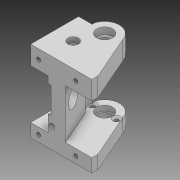
# Autodesk Inventor part: thumb_03 CMC bottom
Saved by Autodesk Inventor 2017 SP1 (Build 210196100, 196)
## iProperties
Created: 2018-02-05
Part Number: thumb_03 CMC bottom
Material: Generic
Document SubType Name: Modeling
Designer: JT
Density: 1 g/cm^3
Appearance: Default
Author: JT
Autodesk Inventor part; units mm, degrees
note: some values were not read from the file. Chosen so that the rebuilt part matches the saved one: direction of "right mount"; direction of "left mount".
sketch3d "geometry"
ref_plane "right inside" through (0, 0, 7.5) normal (0, 0, 1) x (1, 0, 0)
ref_plane "left inside" through (0, 0, -11) normal (0, 0, 1) x (1, 0, 0)
ref_plane "middle top" through (-7.2233, 5.2986, 0) normal (-0.916472, -0.4000988, 0) x (0.4000988, -0.916472, 0)
sketch "Sketch1" plane through (0, 0, 7.5) normal (0, 0, 1) x (1, 0, 0)
  line L0 (-18, 0) -> (5, 0)
  line L1 (5, 0) -> (5, 19)
  line L2 (5, 19) -> (-18, 19)
  line L3 (-18, 19) -> (-18, 0)
  circle A0 centre (-7.6003, 17.4093) radius 5.5
  point P0 (0, 0)
  point P1 (0, 18)
  dimension "d12" = 18
  dimension "d13" = 5
  dimension "d69" = 1
  dimension "d150" = 11
  constraints: 8 end point, 2 parallel, 1 centre point, 1 coincident, 1 horizontal, 1 perpendicular, 1 point on line
  measures "d12" distance from line of point (0, 0) L3
  measures "d13" distance from line of L1 point (0, 0)
  measures "d69" distance from line of L2 point (0, 18)
  measures "d150" diameter of A0
extrude "right" add sketch "Sketch1" along normal blind 7
sketch "Sketch2" plane through (0, 0, -11) normal (0, 0, 1) x (1, 0, 0)
  line L0 (5, 0) -> (-18, 0)
  line L1 (-18, 0) -> (-18, 19)
  line L2 (-18, 19) -> (5, 19)
  line L3 (5, 19) -> (5, 0)
  circle A0 centre (-7.6003, 17.4093) radius 5.5
  point P0 (0, 0)
  point P1 (0, 18)
  dimension "d16" = 18
  dimension "d17" = 5
  dimension "d70" = 1
  dimension "d151" = 11
  constraints: 8 end point, 2 parallel, 1 centre point, 1 coincident, 1 horizontal, 1 perpendicular, 1 point on line
  measures "d16" distance from line of L1 point (0, 0)
  measures "d17" distance from line of point (0, 0) L3
  measures "d70" distance from line of L2 point (0, 18)
  measures "d151" diameter of A0
extrude "left" add sketch "Sketch2" against normal blind 5
sketch "Sketch11" plane through (0, 0, -11) normal (0, 0, 1) x (1, 0, 0)
  line L0 (-0.8483, -9.3042) -> (-15.9776, 25.3514) projected
  line L1 (-12.7683, 18) -> (-19.3151, 18)
  line L2 (-19.3151, 18) -> (-11.457, 0)
  line L3 (-11.457, 0) -> (-4.9101, 0)
  point P0 (0, 0)
  point P1 (0, 18)
  dimension "d66" = 6
  constraints: 6 end point, 4 point on line, 2 parallel, 1 horizontal
  measures "d66" distance between parallel lines of L0 L2
extrude "Extrusion4" add sketch "Sketch11" along normal up to surface (18.5 mm away)
sketch "Sketch4" plane through (0, 0, 7.5) normal (0, 0, 1) x (1, 0, 0)
  point P0 (0, 0)
  point P1 (-7.6003, 17.4093)
hole "thrust bearing pocket" at (-7.6003, 17.4093, 7.5) direction (0, 0, 1) diameter 8.5 depth 3.5
sketch "Sketch7" plane through (0, 0, 7.5) normal (0, 0, 1) x (1, 0, 0)
  point P0 (0, 0)
  point P1 (-7.6003, 17.4093)
hole "worm shaft R" at (-7.6003, 17.4093, 7.5) direction (0, 0, 1) diameter 3.5 end through all
sketch "Sketch5" plane through (0, 0, -11) normal (0, 0, 1) x (1, 0, 0)
  point P0 (0, 0)
  point P1 (-7.6003, 17.4093)
hole "worm shaft L" at (-7.6003, 17.4093, -11) direction (0, 0, -1) diameter 5 end through all counterbore diameter 6 counterbore depth 2
sketch "Sketch6" plane through (-7.2233, 5.2986, 0) normal (-0.916472, -0.4000988, 0) x (0.4000988, -0.916472, 0)
  point P0 (7.746, 0)
  point P1 (0, 0)
hole "CMC bearing" at (-7.2233, 5.2986, 0) direction (-0.916472, -0.4000988, 0) diameter 5 end through all counterbore diameter 7 counterbore depth 2.5
sketch "Sketch9" plane through (0, 0, 14.5) normal (0, 0, 1) x (1, 0, 0)
  point P0 (0, 0)
  point P1 (-7.6003, 17.4093)
hole "Hole5" at (-7.6003, 17.4093, 14.5) direction (0, 0, -1) diameter 6 depth 2.5
ref_plane "clearance angular cut" through (1.9414, 9.2995, 0) normal (-0.916472, -0.4000988, 0) x (0.4000988, -0.916472, 0)
ref_plane "Work Plane4" through (-3.0992, 7.099, 0) normal (-0.916472, -0.4000988, 0) x (0.4000988, -0.916472, 0)
sketch "Sketch12" plane through (0, 0, -11) normal (0, 0, 1) x (1, 0, 0)
  circle A0 centre (-7.6003, 17.4093) radius 5.25
  point P0 (0, 0)
  dimension "d71" = 10.5
  constraints: 1 centre point, 1 coincident
  measures "d71" diameter of A0
extrude "worm cutout" cut sketch "Sketch12" along normal up to surface (18.5 mm away)
sketch "Sketch13" plane through (1.9414, 9.2995, 0) normal (-0.916472, -0.4000988, 0) x (0.4000988, -0.916472, 0)
  line L0 (0, 0) -> (10, 0) construction
  line L1 (0, -25) -> (10, -25)
  line L2 (10, 25) -> (0, 25)
  arc A0 (0, 25) -> (0, -25) centre (0, 0) ccw
  arc A1 (10, -25) -> (10, 25) centre (10, 0) ccw
  point P0 (7.746, 0)
  point P1 (5, 0)
  dimension "d74" = 50
  dimension "d75" = 10
  constraints: 8 end point, 4 point on circle, 4 tangent, 2 centre point, 1 horizontal, 1 midpoint, 1 parallel
  measures "d74" diameter of A1
  measures "d75" horizontal distance of L1.end L0.start
extrude "Extrusion6" cut sketch "Sketch13" against normal through all
ref_plane "Work Plane6" through (3.7744, 10.0997, 0) normal (-0.916472, -0.4000988, 0) x (0.4000988, -0.916472, 0)
split "Split2" [suppressed]
sketch "Sketch14" plane through (-18, 19, -11) normal (0, 1, 0) x (1, 0, 0)
  line L0 (15.7066, 0) -> (15.7066, 5) projected
  line L1 (15.6647, 5) -> (15.7066, 5) projected
  line L2 (0, 0) -> (0, 5) projected
  line L3 (0, -18.5) -> (0, -25.5) projected
  line L4 (5.1348, -25.5) -> (0, -25.5) projected
  line L5 (4.3997, 5) -> (4.3997, 0)
  line L6 (4.3997, -18.5) -> (4.3997, -25.5)
  line L7 (15.7066, -18.5) -> (15.6647, -18.5) projected
  line L8 (5.1348, -18.5) -> (5.1348, -25.5) projected
  line L9 (5.1348, -18.5) -> (0, -18.5) projected
  line L10 (15.7066, -25.5) -> (15.7066, -18.5) projected
  line L11 (15.6647, -25.5) -> (15.6647, -18.5) projected
  line L12 (15.6647, 0) -> (15.7066, 0) projected
  line L13 (5.1348, 5) -> (5.1348, 0) projected
  line L14 (15.6647, 0) -> (15.6647, 5) projected
  line L15 (15.7066, -25.5) -> (15.6647, -25.5) projected
  line L16 (0, 5) -> (5.1348, 5) projected
  line L17 (0, 0) -> (5.1348, 0) projected
  point P0 (18, -11)
  point P1 (10.3997, -11)
  dimension "d80" = 6
  constraints: 4 end point, 2 point on line, 1 collinear
  measures "d80" distance from line of point (10.4, -11) L5
extrude "top cutout" cut sketch "Sketch14" against normal up to surface (1 mm away) contours L2 L16 L5 L17 | L5 L16 L13 L17 | L9 L6 L4 L3 | L9 L8 L4 L6
sketch "Sketch15" plane through (0, 0, -11) normal (0, 0, 1) x (1, 0, 0)
  line L0 (-12.1003, 17.4093) -> (-3.1003, 17.4093) construction
  point P0 (0, 0)
  point P1 (-7.6003, 17.4093)
  point P2 (-7.6003, 17.4093)
  dimension "d83" = 9
  constraints: 2 end point, 1 coincident, 1 horizontal, 1 midpoint
  measures "d83" distance of L0.end L0.start
hole "motor mount" at (-12.1003, 17.4093, -11) at (-3.1003, 17.4093, -11) direction (0, 0, -1) diameter 1.6 end through all countersink diameter 3 countersink angle 90
sketch "Sketch16" plane through (-19.3151, 18, -11) normal (0, 1, 0) x (1, 0, 0)
  line L0 (6.4982, -18.5) -> (6.4982, 0) projected
  line L1 (5.8361, 0) -> (6.4982, 0) projected
  line L2 (1.3151, 5) -> (6.4499, 5) projected
  line L3 (1.3151, 0) -> (1.3151, 5) projected
  line L4 (0, 0) -> (1.3151, 0) projected
  line L5 (0, 0) -> (0, -18.5) projected
  line L6 (0, -18.5) -> (1.3151, -18.5) projected
  line L7 (1.3151, -25.5) -> (1.3151, -18.5) projected
  line L8 (6.4499, -25.5) -> (1.3151, -25.5) projected
  line L9 (6.4982, -18.5) -> (6.4499, -18.5) projected
  line L10 (1.3151, 2.5) -> (5.7149, 2.5) construction
  line L11 (1.3151, -22) -> (5.7149, -22) construction
  line L12 (0, -9.25) -> (6.4982, -9.25) construction
  line L13 (6.4499, -18.5) -> (6.4499, -25.5) projected
  line L14 (6.4499, 5) -> (6.4499, 0.5335) projected
  point P0 (19.3151, -11)
  point P1 (3.515, 2.5)
  point P2 (4.9982, -2.75)
  point P3 (4.9982, -15.75)
  point P4 (3.515, -22)
  point P5 (3.515, 2.5)
  point P6 (3.515, -22)
  dimension "d91" = 1.5
  dimension "d92" = 13
  constraints: 6 end point, 6 midpoint, 2 coincident, 1 symmetric about line, 1 other
  measures "d91" distance from line of L0 point (4.998, -2.75)
  measures "d92" distance of point (4.998, -15.75) point (4.998, -2.75)
hole "top mount" at (-15.8001, 18, -13.5) at (-15.8001, 18, 11) direction (0, -1, 0) diameter 1.567 depth 6.3 tip angle 118 thread size "M2x0.4" class "6H" standard "ANSI Metric M Profile"
sketch "Sketch25" plane through (-19.3151, 18, -11) normal (0, 1, 0) x (1, 0, 0)
  point P0 (19.3151, -11)
  point P1 (4.9982, -15.75)
  point P2 (4.9982, -2.75)
hole "top mount screws" at (-14.3169, 18, 4.75) at (-14.3169, 18, -8.25) direction (0, -1, 0) diameter 2 depth 5
sketch "Sketch17" plane through (0, 0, 14.5) normal (0, 0, 1) x (1, 0, 0)
  line L0 (-0.5303, -10.0324) -> (-17.8852, 29.7208) projected
  line L1 (-14.2665, 16.4331) -> (-8.2335, 2.6139) construction
  point P0 (0, 0)
  point P1 (0, 18)
  point P2 (-11.0215, 9)
  dimension "d100" = 2
  dimension "d101" = 9
  constraints: 2 end point, 1 parallel, 1 point on line
  measures "d100" distance between parallel lines of L0 L1
  measures "d101" vertical distance of point (-11.021, 9) point (0, 18)
hole "right mount" at (-11.0215, 9, 14.5) direction (0, 0, -1) diameter 2.2 depth 7 counterbore diameter 4 counterbore depth 2
sketch "Sketch18" plane through (0, 0, -16) normal (0, 0, -1) x (-1, 0, 0)
  line L0 (4.9101, 0) -> (10.6425, 13.1306) projected
  line L1 (10.6425, 13.1306) -> (4.9101, 0) projected
  line L2 (5.8229, 2.0909) -> (8.6236, 8.5062) projected
  line L3 (4.9157, -4.986) -> (12.5315, 12.4589) construction
  point P0 (0, 0)
  point P1 (11.0215, 9)
  point P2 (0, 18)
  dimension "d110" = 2
  dimension "d111" = 9
  constraints: 2 end point, 1 parallel, 1 point on line
  measures "d110" distance between parallel lines of L3 L0
  measures "d111" vertical distance of point (11.021, 9) point (0, 18)
hole "left mount" at (-11.0215, 9, -16) direction (0, 0, 1) diameter 2.2 depth 5 counterbore diameter 4 counterbore depth 2
sketch "Sketch19" plane through (-18, 0, 14.5) normal (0, -1, 0) x (1, 0, 0)
  line L0 (0, -7) -> (6.543, -7) projected
  line L1 (6.543, -25.5) -> (6.543, -7) projected
  line L2 (6.543, -25.5) -> (0, -25.5) projected
  line L3 (0, -25.5) -> (0, -30.5) projected
  line L4 (23, -30.5) -> (0, -30.5) projected
  line L5 (23, -25.5) -> (23, -30.5) projected
  line L6 (23, -25.5) -> (13.0899, -25.5) projected
  line L7 (13.0899, -25.5) -> (13.0899, -7) projected
  line L8 (13.0899, -7) -> (23, -7) projected
  line L9 (23, -7) -> (23, 0) projected
  line L10 (0, 0) -> (23, 0) projected
  line L11 (0, -7) -> (0, 0) projected
  line L12 (23, -28) -> (0, -28) construction
  line L13 (23, -3.5) -> (0, -3.5) construction
  line L14 (13.0899, -16.25) -> (6.543, -16.25) construction
  point P0 (18, -14.5)
  point P1 (17, -28)
  point P2 (3, -28)
  point P3 (17, -3.5)
  point P4 (3, -3.5)
  point P5 (8.043, -22.75)
  dimension "d119" = 6
  dimension "d120" = 3
  dimension "d121" = 3
  dimension "d122" = 6
  dimension "d124" = 1.5
  dimension "d173" = 6.5
  constraints: 6 end point, 6 midpoint, 4 point on line
  measures "d119" distance from line of point (17, -28) L5
  measures "d120" distance of L12.end point (3, -28)
  measures "d121" distance from line of L11 point (3, -3.5)
  measures "d122" distance from line of point (17, -3.5) L9
  measures "d124" distance from line of L1 point (8.043, -22.75)
  measures "d173" distance from line of L14 point (8.043, -22.75)
hole "bottom mount" at (-1, 0, -13.5) at (-15, 0, -13.5) at (-1, 0, 11) at (-15, 0, 11) direction (0, 1, 0) diameter 1.567 depth 8.5 tip angle 118 thread size "M2x0.4" class "6H" standard "ANSI Metric M Profile"
sketch "Sketch24" plane through (-18, 0, 14.5) normal (0, -1, 0) x (1, 0, 0)
  point P0 (18, -14.5)
  point P1 (8.043, -22.75)
hole "bottom mount screw" at (-9.957, 0, -8.25) direction (0, 1, 0) diameter 2 depth 8
hole "right thread" at (-11.0215, 9, 7.5) direction (0, 0, -1) diameter 2 depth 7.3
hole "left thread" at (-11.0215, 9, -11) direction (0, 0, 1) diameter 2 depth 7.3 tip angle 118
sketch "Sketch20" plane through (-3.0992, 7.099, 0) normal (-0.916472, -0.4000988, 0) x (0.4000988, -0.916472, 0)
  circle A0 centre (0, 0) radius 8.5
  point P0 (7.746, 0)
  point P1 (0, 0)
  dimension "d156" = 17
  constraints: 1 centre point, 1 coincident
  measures "d156" diameter of A0
extrude "wormgear pocket" cut sketch "Sketch20" along normal mid plane 5
sketch "Sketch21" plane through (-19.3151, 18, -11) normal (-0.916472, -0.4000988, 0) x (0, 0, 1)
  arc A0 (5, -16.4784) -> (17, -16.4784) centre (11, -16.4784) ccw
  line L0 (5, -16.4784) -> (5, -6.4784)
  line L1 (5, -6.4784) -> (17, -6.4784)
  line L2 (17, -6.4784) -> (17, -16.4784)
  point P0 (11, -24.2245)
  dimension "d159" = 12
  dimension "d160" = 10
  constraints: 6 end point, 2 point on circle, 2 tangent, 2 vertical, 1 centre point, 1 coincident, 1 perpendicular
  measures "d159" diameter of A0
  measures "d160" distance from line of point (11, -16.478) L1
extrude "angle sensor" cut sketch "Sketch21" against normal blind 1
sketch "Sketch22" plane through (-18.3987, 18.4001, -11) normal (-0.916472, -0.4000988, 0) x (0, 0, 1)
  line L0 (8.5, -11.9784) -> (13.5, -11.9784) construction
  line L1 (13.5, -11.9784) -> (13.5, -19.4784) construction
  line L2 (13.5, -19.4784) -> (8.5, -19.4784) construction
  line L3 (8.5, -19.4784) -> (8.5, -11.9784) construction
  line L4 (8.5, -11.9784) -> (13.5, -19.4784) construction
  line L5 (13.5, -11.9784) -> (8.5, -19.4784) construction
  point P0 (11, -24.2245)
  point P1 (11, -16.4784)
  point P2 (11, -15.7284)
  dimension "d163" = 5
  dimension "d164" = 7.5
  dimension "d165" = 4.5
  constraints: 12 end point, 2 midpoint, 2 parallel, 1 horizontal, 1 perpendicular, 1 vertical alignment
  measures "d163" distance between parallel lines of L1 L3
  measures "d164" distance between parallel lines of L2 L0
  measures "d165" distance from line of point (11, -16.478) L0
hole "Hole13" at (-11.8057, 3.2981, 0) at (-13.6061, 7.4222, -2.5) at (-13.6061, 7.4222, 2.5) at (-10.6054, 0.5486, 2.5) at (-10.6054, 0.5486, -2.5) direction (0.916472, 0.4000988, 0) diameter 1 depth 1.5 tip angle 118
sketch "Sketch23" plane through (-19.3151, 18, -11) normal (-0.916472, -0.4000988, 0) x (0, 0, 1)
  line L0 (0, 11.5711) -> (0, -37.9321) projected
  point P0 (11, -24.2245)
  point P1 (2.5, -9.4784)
  point P2 (2.5, -15.4784)
  point P3 (11, -16.4784)
  dimension "d174" = 2.5
  dimension "d175" = 6
  dimension "d176" = 1
  constraints: 1 vertical alignment
  measures "d174" distance from line of point (2.5, -9.478) L0
  measures "d175" distance of point (2.5, -15.478) point (2.5, -9.478)
  measures "d176" vertical distance of point (11, -16.478) point (2.5, -15.478)
hole "Hole14" at (-15.5228, 9.3133, -8.5) at (-13.1222, 3.8144, -8.5) at (-12.7221, 2.898, 0) direction (0.916472, 0.4000988, 0) diameter 1.22 depth 2 tip angle 118
equation "\"d46\" = thumb_axis_beta_local"
equation "\"thumb_axis_beta_local\" = thumb_axis_beta"
body "Solid1"
